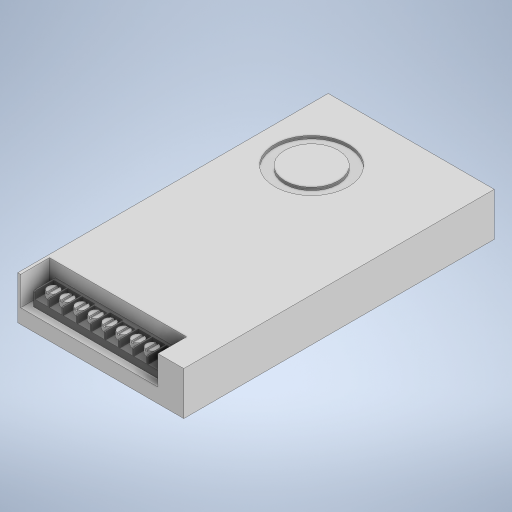
# Autodesk Inventor part: 24v_Tapmásikamianagyobb
Saved by Autodesk Inventor 2023 (Build 270158000, 158)
## iProperties
Created: 2023-04-10
Part Number: 24v_Tapmásikamianagyobb
Material: Generic
Document SubType Name: Modeling
Designer: nagyb
Density: 1 g/cm^3
Appearance: Default
Author: nagyb
Autodesk Inventor part; units mm, degrees
ref_plane "YZ Plane" through (0, 0, 0) normal (1, 0, 0) x (0, 1, 0)
ref_plane "XZ Plane" through (0, 0, 0) normal (0, 1, 0) x (-1, 0, 0)
ref_plane "XY Plane" through (0, 0, 0) normal (0, 0, 1) x (1, 0, 0)
sketch "Sketch1" plane through (0, 0, 0) normal (0, 1, 0) x (-1, 0, 0)
  line L0 (57.5, 107.5) -> (-57.5, 107.5)
  line L1 (-57.5, 107.5) -> (-57.5, -107.5)
  line L2 (-57.5, -107.5) -> (57.5, -107.5)
  line L3 (57.5, -107.5) -> (57.5, 107.5)
  line L4 (57.5, 107.5) -> (-57.5, -107.5) construction
  line L5 (-57.5, 107.5) -> (57.5, -107.5) construction
  point P0 (0, 0)
  dimension "d0" = 215
  dimension "d1" = 115
  constraints: 12 end point, 2 midpoint, 2 parallel, 1 horizontal, 1 perpendicular
  measures "d0" distance of L2.end L0.start
  measures "d1" distance of L1.end L2.end
extrude "Extrusion1" add sketch "Sketch1" along normal blind 30
sketch "Sketch2" plane through (0, 30, 0) normal (0, 1, 0) x (1, 0, 0)
  line L0 (-57.5, -107.5) -> (57.5, -107.5) projected
  line L1 (-55.5, -107.5) -> (39.5, -107.5)
  line L2 (39.5, -107.5) -> (39.5, -87.5)
  line L3 (39.5, -87.5) -> (-55.5, -87.5)
  line L4 (-55.5, -87.5) -> (-55.5, -107.5)
  line L5 (-57.5, 107.5) -> (-57.5, -107.5) projected
  point P0 (0, 0)
  dimension "d4" = 95
  dimension "d5" = 20
  dimension "d6" = 2
  constraints: 8 end point, 2 parallel, 1 horizontal, 1 perpendicular, 1 point on line
  measures "d4" distance of L2.end L3.end
  measures "d5" distance of L3.end L1.start
  measures "d6" distance between parallel lines of L5 L4
extrude "Extrusion2" cut sketch "Sketch2" against normal blind 20
sketch "Sketch3" plane through (0, 10, 0) normal (0, 1, 0) x (1, 0, 0)
  line L0 (-55.5, -87.5) -> (39.5, -87.5) projected
  line L1 (-51.5, -87.5) -> (38.5, -87.5)
  line L2 (38.5, -87.5) -> (38.5, -102.5)
  line L3 (38.5, -102.5) -> (-51.5, -102.5)
  line L4 (-51.5, -102.5) -> (-51.5, -87.5)
  line L5 (39.5, -87.5) -> (39.5, -107.5) projected
  point P0 (0, 0)
  dimension "d9" = 90
  dimension "d10" = 15
  dimension "d11" = 1
  constraints: 8 end point, 2 parallel, 1 horizontal, 1 perpendicular, 1 point on line
  measures "d9" distance of L2.end L3.end
  measures "d10" distance of L3.end L1.start
  measures "d11" distance between parallel lines of L5 L2
extrude "Extrusion3" add sketch "Sketch3" along normal blind 10
fillet "Fillet1" radius 1 1 edges at (-6.5, 20, 102.5)
sketch "Sketch4" plane through (0, 20, 0) normal (0, 1, 0) x (1, 0, 0)
  line L0 (38.5, -102.5) -> (-51.5, -102.5) projected
  line L1 (-50.5, -89.5) -> (-41.7, -89.5)
  line L2 (-41.7, -89.5) -> (-41.7, -102.5)
  line L3 (-41.7, -102.5) -> (-50.5, -102.5)
  line L4 (-50.5, -102.5) -> (-50.5, -89.5)
  line L5 (-51.5, -87.5) -> (-51.5, -101.5) projected
  line L6 (-55.5, -87.5) -> (39.5, -87.5) projected
  line L7 (-40.7, -89.5) -> (-31.9, -89.5)
  line L8 (-31.9, -89.5) -> (-31.9, -102.5)
  line L9 (-31.9, -102.5) -> (-40.7, -102.5)
  line L10 (-40.7, -102.5) -> (-40.7, -89.5)
  line L11 (-30.9, -89.5) -> (-22.1, -89.5)
  line L12 (-22.1, -89.5) -> (-22.1, -102.5)
  line L13 (-22.1, -102.5) -> (-30.9, -102.5)
  line L14 (-30.9, -102.5) -> (-30.9, -89.5)
  line L15 (-21.1, -90.6883) -> (-12.3, -90.6883)
  line L16 (-12.3, -90.6883) -> (-12.3, -102.5)
  line L17 (-12.3, -102.5) -> (-21.1, -102.5)
  line L18 (-21.1, -102.5) -> (-21.1, -90.6883)
  line L19 (-11.4956, -89.5) -> (-2.6956, -89.5)
  line L20 (-2.6956, -89.5) -> (-2.6956, -102.5)
  line L21 (-2.6956, -102.5) -> (-11.4956, -102.5)
  line L22 (-11.4956, -102.5) -> (-11.4956, -89.5)
  line L23 (-1.6956, -90.6883) -> (7.1044, -90.6883)
  line L24 (7.1044, -90.6883) -> (7.1044, -102.5)
  line L25 (7.1044, -102.5) -> (-1.6956, -102.5)
  line L26 (-1.6956, -102.5) -> (-1.6956, -90.6883)
  line L27 (8.1044, -89.5) -> (16.9044, -89.5)
  line L28 (16.9044, -89.5) -> (16.9044, -102.5)
  line L29 (16.9044, -102.5) -> (8.1044, -102.5)
  line L30 (8.1044, -102.5) -> (8.1044, -89.5)
  line L31 (17.9044, -89.5) -> (26.7044, -89.5)
  line L32 (26.7044, -89.5) -> (26.7044, -102.5)
  line L33 (26.7044, -102.5) -> (17.9044, -102.5)
  line L34 (17.9044, -102.5) -> (17.9044, -89.5)
  line L35 (27.7044, -89.5) -> (36.5044, -89.5)
  line L36 (36.5044, -89.5) -> (36.5044, -102.5)
  line L37 (36.5044, -102.5) -> (27.7044, -102.5)
  line L38 (27.7044, -102.5) -> (27.7044, -89.5)
  point P0 (0, 0)
  point P1 (-22.1, -96)
  point P2 (-26.5, -89.5)
  point P3 (-12.3, -96.5941)
  point P4 (-11.4956, -96)
  point P5 (-7.0956, -89.5)
  point P6 (16.9044, -96)
  point P7 (8.1044, -96)
  point P8 (17.9044, -96)
  point P9 (8.1044, -102.5)
  point P10 (-1.6956, -102.5)
  point P11 (-11.4956, -102.5)
  point P12 (-30.9, -102.5)
  point P13 (-40.7, -102.5)
  point P14 (-50.5, -102.5)
  dimension "d15" = 1
  dimension "d16" = 2
  dimension "d17" = 8.8
  dimension "d18" = 2
  dimension "d19" = 1
  dimension "d20" = 8.8
  dimension "d21" = 1
  dimension "d22" = 8.8
  dimension "d23" = 2
  dimension "d24" = 1
  dimension "d25" = 8.8
  dimension "d26" = 8.8
  dimension "d27" = 1
  dimension "d28" = 2
  dimension "d29" = 8.8
  dimension "d30" = 1
  dimension "d31" = 1
  dimension "d32" = 8.8
  dimension "d33" = 1
  dimension "d34" = 8.8
  dimension "d35" = 1
  dimension "d36" = 8.8
  dimension "d37" = 2
  constraints: 72 end point, 18 parallel, 9 horizontal, 9 perpendicular, 8 midpoint, 1 point on line, 10 other
  measures "d15" distance between parallel lines of L4 L5
  measures "d16" distance between parallel lines of L6 L1
  measures "d17" distance between parallel lines of L2 L4
  measures "d18" distance between parallel lines of L6 L7
  measures "d19" distance between parallel lines of L2 L10
  measures "d20" distance between parallel lines of L8 L10
  measures "d21" distance between parallel lines of L8 L14
  measures "d22" distance from line of point (-22.1, -96) L14
  measures "d23" distance from line of point (-26.5, -89.5) L6
  measures "d24" distance between parallel lines of L18 L12
  measures "d25" distance between parallel lines of L18 L16
  measures "d26" distance of L19.start L19.end
  measures "d27" distance of point (-12.3, -96.594) point (-11.496, -96)
  measures "d28" distance from line of L6 point (-7.096, -89.5)
  measures "d29" distance of L23.start L23.end
  measures "d30" distance between parallel lines of L20 L26
  measures "d31" distance between parallel lines of L24 L30
  measures "d32" distance of point (16.904, -96) point (8.104, -96)
  measures "d33" distance of point (16.904, -96) point (17.904, -96)
  measures "d34" distance between parallel lines of L32 L34
  measures "d35" distance between parallel lines of L38 L32
  measures "d36" distance between parallel lines of L38 L36
  measures "d37" distance between parallel lines of L6 L35
extrude "Extrusion4" cut sketch "Sketch4" against normal blind 5
sketch "Sketch5" plane through (0, 15, 0) normal (0, 1, 0) x (1, 0, 0)
  circle A0 centre (-46.1, -94.216) radius 4
  circle A1 centre (-36.3, -94.216) radius 4
  line L0 (-50.5, -101.5) -> (-50.5, -89.5) projected
  line L1 (-40.7, -101.5) -> (-40.7, -89.5) projected
  circle A2 centre (-26.5, -94.216) radius 4
  line L2 (-30.9, -101.5) -> (-30.9, -89.5) projected
  circle A3 centre (-16.7, -94.216) radius 4
  line L3 (-21.1, -101.5) -> (-21.1, -90.6883) projected
  circle A4 centre (-7.0956, -94.216) radius 4
  line L4 (-11.4956, -101.5) -> (-11.4956, -89.5) projected
  circle A5 centre (2.7044, -94.216) radius 4
  circle A6 centre (12.5044, -94.216) radius 4
  circle A7 centre (22.3044, -94.216) radius 4
  circle A8 centre (32.1044, -94.216) radius 4
  line L5 (-1.6956, -101.5) -> (-1.6956, -90.6883) projected
  line L6 (8.1044, -101.5) -> (8.1044, -89.5) projected
  line L7 (17.9044, -101.5) -> (17.9044, -89.5) projected
  line L8 (27.7044, -101.5) -> (27.7044, -89.5) projected
  point P0 (0, 0)
  dimension "d40" = 4.4
  dimension "d41" = 4.4
  dimension "d42" = 8
  dimension "d43" = 8
  dimension "d44" = 8
  dimension "d45" = 4.4
  dimension "d46" = 4.4
  dimension "d47" = 8
  dimension "d48" = 4.4
  dimension "d49" = 8
  dimension "d50" = 4.4
  dimension "d51" = 8
  dimension "d52" = 4.4
  dimension "d53" = 8
  dimension "d54" = 4.4
  dimension "d55" = 8
  dimension "d56" = 4.4
  dimension "d57" = 8
  constraints: 9 centre point
  measures "d40" distance from line of L0 A0.centre
  measures "d41" distance from line of A1.centre L1
  measures "d42" diameter of A0
  measures "d43" diameter of A1
  measures "d44" diameter of A2
  measures "d45" distance from line of L2 A2.centre
  measures "d46" distance from line of A3.centre L3
  measures "d47" diameter of A3
  measures "d48" distance from line of L4 A4.centre
  measures "d49" diameter of A4
  measures "d50" distance from line of L5 A5.centre
  measures "d51" diameter of A5
  measures "d52" distance from line of L6 A6.centre
  measures "d53" diameter of A6
  measures "d54" distance from line of L7 A7.centre
  measures "d55" diameter of A7
  measures "d56" distance from line of L8 A8.centre
  measures "d57" diameter of A8
extrude "Extrusion5" add sketch "Sketch5" along normal blind 4
sketch "Sketch6" plane through (-46.1, 19, 94.216) normal (0, 1, 0) x (1, 0, 0)
  line L0 (0.75, -4.0442) -> (-0.75, -4.0442)
  line L1 (-0.75, -4.0442) -> (-0.75, 4.0442)
  line L2 (-0.75, 4.0442) -> (0.75, 4.0442)
  line L3 (0.75, 4.0442) -> (0.75, -4.0442)
  circle A0 centre (0, 0) radius 4 projected
  line L4 (0.75, -4.0442) -> (-0.75, 4.0442) construction
  line L5 (-0.75, -4.0442) -> (0.75, 4.0442) construction
  point P0 (46.1, 94.216)
  dimension "d60" = 1.5
  constraints: 12 end point, 2 midpoint, 2 parallel, 1 horizontal, 1 perpendicular
  measures "d60" distance between parallel lines of L3 L1
sketch "Sketch7" plane through (-36.3, 19, 94.216) normal (0, 1, 0) x (1, 0, 0)
  line L0 (0.75, -4.4194) -> (-0.75, -4.4194)
  line L1 (-0.75, -4.4194) -> (-0.75, 4.0806)
  line L2 (-0.75, 4.0806) -> (0.75, 4.0806)
  line L3 (0.75, 4.0806) -> (0.75, -4.4194)
  line L4 (0.75, -3.5641) -> (-0.75, 3.5713) construction
  line L5 (-0.75, -3.5641) -> (0.75, 3.5713) construction
  point P0 (36.3, 94.216)
  point P1 (0, 0.0036)
  dimension "d61" = 1.5
  dimension "d62" = 8.5
  constraints: 12 end point, 2 midpoint, 2 parallel, 1 horizontal, 1 perpendicular
  measures "d61" distance between parallel lines of L3 L1
  measures "d62" distance of L0.end L1.end
sketch "Sketch8" plane through (-26.5, 19, 94.216) normal (0, 1, 0) x (1, 0, 0)
  line L0 (0.75, -4.1692) -> (-0.75, -4.1692)
  line L1 (-0.75, -4.1692) -> (-0.75, 4.0308)
  line L2 (-0.75, 4.0308) -> (0.75, 4.0308)
  line L3 (0.75, 4.0308) -> (0.75, -4.1692)
  line L4 (0.75, -2.9359) -> (-0.75, 5.0641) construction
  line L5 (-0.75, -2.9359) -> (0.75, 5.0641) construction
  point P0 (26.5, 94.216)
  point P1 (0, 1.0641)
  dimension "d63" = 1.5
  dimension "d64" = 8.2
  constraints: 12 end point, 2 midpoint, 2 parallel, 1 horizontal, 1 perpendicular
  measures "d63" distance between parallel lines of L3 L1
  measures "d64" distance of L0.end L1.end
extrude "Extrusion6" cut sketch "Sketch6" against normal blind 1 contours L0 L1 A0 L3 | A0 L1 L3 | A0 L1 L2 L3
extrude "Extrusion7" cut sketch "Sketch7" against normal blind 1
extrude "Extrusion8" cut sketch "Sketch8" against normal blind 1
sketch "Sketch9" plane through (-16.7, 19, 94.216) normal (0, 1, 0) x (1, 0, 0)
  line L0 (0.7517, -4.1161) -> (-0.7483, -4.1161)
  line L1 (-0.7483, -4.1161) -> (-0.7483, 4.0839)
  line L2 (-0.7483, 4.0839) -> (0.7517, 4.0839)
  line L3 (0.7517, 4.0839) -> (0.7517, -4.1161)
  line L4 (0.3696, -1.4172) -> (-1.1304, 4.335) construction
  line L5 (-1.1304, -1.4172) -> (0.3696, 4.335) construction
  point P0 (16.7, 94.216)
  point P1 (-0.3804, 1.4589)
  dimension "d71" = 1.5
  dimension "d72" = 8.2
  constraints: 12 end point, 2 midpoint, 2 parallel, 1 horizontal, 1 perpendicular
  measures "d71" distance of L1.end L2.end
  measures "d72" distance of L2.end L0.start
extrude "Extrusion9" cut sketch "Sketch9" against normal blind 1
sketch "Sketch10" plane through (-7.0956, 19, 94.216) normal (0, 1, 0) x (1, 0, 0)
  line L0 (0.743, -4.2555) -> (-0.757, -4.2555)
  line L1 (-0.757, -4.2555) -> (-0.757, 4.3351)
  line L2 (-0.757, 4.3351) -> (0.743, 4.3351)
  line L3 (0.743, 4.3351) -> (0.743, -4.2555)
  line L4 (0.743, -4.2555) -> (-0.757, 4.3351) construction
  line L5 (-0.757, -4.2555) -> (0.743, 4.3351) construction
  point P0 (7.0956, 94.216)
  point P1 (-0.007, 0.0398)
  dimension "d75" = 1.5
  constraints: 12 end point, 2 midpoint, 2 parallel, 1 horizontal, 1 perpendicular
  measures "d75" distance of L1.end L2.end
extrude "Extrusion10" cut sketch "Sketch10" against normal blind 1
sketch "Sketch11" plane through (2.7044, 19, 94.216) normal (0, 1, 0) x (1, 0, 0)
  line L0 (0.7237, -4.0227) -> (-0.7763, -4.0227)
  line L1 (-0.7763, -4.0227) -> (-0.7763, 4.3147)
  line L2 (-0.7763, 4.3147) -> (0.7237, 4.3147)
  line L3 (0.7237, 4.3147) -> (0.7237, -4.0227)
  line L4 (0.7237, -4.0227) -> (-0.7763, 4.3147) construction
  line L5 (-0.7763, -4.0227) -> (0.7237, 4.3147) construction
  point P0 (-2.7044, 94.216)
  point P1 (-0.0263, 0.146)
  dimension "d78" = 1.5
  constraints: 12 end point, 2 midpoint, 2 parallel, 1 horizontal, 1 perpendicular
  measures "d78" distance of L1.end L2.end
extrude "Extrusion11" cut sketch "Sketch11" against normal blind 1
sketch "Sketch12" plane through (12.5044, 19, 94.216) normal (0, 1, 0) x (1, 0, 0)
  line L0 (0.7314, -4.1412) -> (-0.7686, -4.1412)
  line L1 (-0.7686, -4.1412) -> (-0.7686, 4.3518)
  line L2 (-0.7686, 4.3518) -> (0.7314, 4.3518)
  line L3 (0.7314, 4.3518) -> (0.7314, -4.1412)
  line L4 (0.7314, -4.1412) -> (-0.7686, 4.3518) construction
  line L5 (-0.7686, -4.1412) -> (0.7314, 4.3518) construction
  point P0 (-12.5044, 94.216)
  point P1 (-0.0186, 0.1053)
  dimension "d81" = 1.5
  constraints: 12 end point, 2 midpoint, 2 parallel, 1 horizontal, 1 perpendicular
  measures "d81" distance of L1.end L2.end
extrude "Extrusion12" cut sketch "Sketch12" against normal blind 1
sketch "Sketch13" plane through (22.3044, 19, 94.216) normal (0, 1, 0) x (1, 0, 0)
  line L0 (0.6965, -4.0732) -> (-0.8035, -4.0732)
  line L1 (-0.8035, -4.0732) -> (-0.8035, 4.0912)
  line L2 (-0.8035, 4.0912) -> (0.6965, 4.0912)
  line L3 (0.6965, 4.0912) -> (0.6965, -4.0732)
  line L4 (0.6965, -3.7541) -> (-0.8035, 4.3306) construction
  line L5 (-0.8035, -3.7541) -> (0.6965, 4.3306) construction
  point P0 (-22.3044, 94.216)
  point P1 (-0.0535, 0.2882)
  dimension "d84" = 1.5
  constraints: 12 end point, 2 midpoint, 2 parallel, 1 horizontal, 1 perpendicular
  measures "d84" distance of L1.end L2.end
extrude "Extrusion13" cut sketch "Sketch13" against normal blind 1
sketch "Sketch14" plane through (32.1044, 19, 94.216) normal (0, 1, 0) x (1, 0, 0)
  line L0 (0.7632, -4.5901) -> (-0.7368, -4.5901)
  line L1 (-0.7368, -4.5901) -> (-0.7368, 4.4317)
  line L2 (-0.7368, 4.4317) -> (0.7632, 4.4317)
  line L3 (0.7632, 4.4317) -> (0.7632, -4.5901)
  line L4 (0.7632, -4.5901) -> (-0.7368, 4.4317) construction
  line L5 (-0.7368, -4.5901) -> (0.7632, 4.4317) construction
  point P0 (-32.1044, 94.216)
  point P1 (0.0132, -0.0792)
  dimension "d87" = 1.5
  constraints: 12 end point, 2 midpoint, 2 parallel, 1 horizontal, 1 perpendicular
  measures "d87" distance of L1.end L2.end
extrude "Extrusion14" cut sketch "Sketch14" against normal blind 1
sketch "Sketch15" plane through (0, 30, 0) normal (0, 1, 0) x (1, 0, 0)
  circle A0 centre (-20, 58.5) radius 25.5
  line L0 (-57.5, 107.5) -> (-57.5, -107.5) projected
  line L1 (57.5, 107.5) -> (-57.5, 107.5) projected
  line L2 (-57.5, -107.5) -> (57.5, -107.5) projected
  circle A1 centre (-20, 58.5) radius 18.4524
  point P0 (0, 0)
  point P1 (-55.5, -107.5)
  constraints: 2 centre point, 1 coincident
extrude "Extrusion15" cut sketch "Sketch15" against normal blind 2
body "Solid1"
